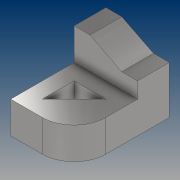
# Autodesk Inventor part: 37
Saved by Autodesk Inventor 2020.2 (Build 242310000, 310)
## iProperties
Created: 2020-09-17
Part Number: 37
Material: 鋼、碳鋼
Document SubType Name: Modeling
Designer: user
Density: 7.85 g/cm^3
Appearance: 半拋光
Mass: 426.123 g
Surface Area: 112.695 cm^2
Volume: 54.2832 cm^3
Author: user
Autodesk Inventor part; units mm, degrees
ref_plane "YZ Plane" through (0, 0, 0) normal (1, 0, 0) x (0, 1, 0)
ref_plane "XZ Plane" through (0, 0, 0) normal (0, 1, 0) x (-1, 0, 0)
ref_plane "XY Plane" through (0, 0, 0) normal (0, 0, 1) x (1, 0, 0)
sketch "草圖1" plane through (0, 0, 0) normal (0, 1, 0) x (-1, 0, 0)
  line L0 (20, 0) -> (-20, 0)
  line L1 (-20, 0) -> (-20, 60)
  line L2 (-20, 60) -> (20, 60)
  line L3 (20, 60) -> (20, 0)
  point P0 (0, 0)
  point P1 (0, 0)
  dimension "d0" = 40
  dimension "d1" = 60
  constraints: 8 end point, 2 parallel, 1 coincident, 1 horizontal, 1 midpoint, 1 perpendicular
  measures "d0" distance of L1.end L2.end
  measures "d1" distance of L2.end L0.start
extrude "擠出1" add sketch "草圖1" along normal blind 40
sketch "草圖2" plane through (20, 0, 60) normal (1, 0, 0) x (0, 0, -1)
  line L0 (60, 40) -> (60, 0) projected
  line L1 (60, 0) -> (0, 0) projected
  line L2 (0, 0) -> (0, 40) projected
  line L3 (0, 40) -> (60, 40) projected
  line L4 (-24.1711, 57.1186) -> (40, 57.1186)
  line L5 (40, 57.1186) -> (40, 20)
  line L6 (40, 20) -> (-24.1711, 20)
  line L7 (-24.1711, 20) -> (-24.1711, 57.1186)
  dimension "d4" = 40
  dimension "d5" = 20
  constraints: 8 end point, 2 parallel, 1 horizontal, 1 perpendicular
  measures "d4" distance between parallel lines of L5 L2
  measures "d5" distance between parallel lines of L6 L3
extrude "擠出2" cut sketch "草圖2" against normal through all contours L5 L6 L2 L3 | L3 L2 L6 L7 L4 L5
sketch "草圖3" plane through (20, 20, 20) normal (0, 0, 1) x (1, 0, 0)
  line L0 (-40, 20) -> (0, 20) projected
  line L1 (0, 20) -> (0, 0) projected
  line L2 (-40, 0) -> (0, 0) projected
  line L3 (-40, -20) -> (-40, 0) projected
  line L4 (0, -20) -> (-40, -20) projected
  line L5 (0, 0) -> (0, -20) projected
  line L6 (-40, 0) -> (-40, 20) projected
  line L7 (0, 20) -> (-40, 20) projected
  line L8 (-30, 20) -> (-10, 10)
  line L9 (-10, 10) -> (0, 10)
  line L10 (0, -20) -> (0, 20) projected
  point P0 (-20, -20)
  point P1 (0, 10)
  dimension "d8" = 10
  dimension "d9" = 10
  dimension "d10" = 10
  constraints: 4 end point, 2 point on line, 1 perpendicular
  measures "d8" distance between parallel lines of L2 L9
  measures "d9" distance from line of L8.start L6
  measures "d10" distance of L8.end L9.end
extrude "擠出3" cut sketch "草圖3" against normal through all contours L0 L1 L9 L8
sketch "草圖4" plane through (20, 20, 60) normal (0, 1, 0) x (1, 0, 0)
  line L0 (0, 60) -> (0, 40) projected
  line L1 (0, 40) -> (0, 0) projected
  line L2 (0, 0) -> (-40, 0) projected
  line L3 (-40, 0) -> (-40, 40) projected
  line L4 (-40, 40) -> (-40, 60) projected
  line L5 (-40, 60) -> (0, 60) projected
  line L6 (0, 40) -> (-40, 40) projected
  line L7 (-30, 30) -> (-30, 10)
  line L8 (-30, 10) -> (-10, 30)
  line L9 (-10, 30) -> (-30, 30)
  point P0 (-20, 60)
  dimension "d13" = 20
  dimension "d14" = 10
  dimension "d15" = 10
  constraints: 6 end point, 2 perpendicular, 1 vertical
  measures "d13" distance of L7.start L7.end
  measures "d14" distance between parallel lines of L7 L3
  measures "d15" distance between parallel lines of L6 L9
extrude "擠出4" cut sketch "草圖4" against normal through all contours L9 L8 L7
fillet "圓角1" radius 20 1 edges at (20, 10, 60)
